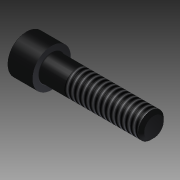
# Autodesk Inventor part: 3071
Saved by Autodesk Inventor 2016 (Build 200138000, 138)
## iProperties
Category: PARTsolutions
Company: 8020
Created: 2016-04-17
Part Number: 3071
Catalog Web Link: www.cadenas.de
Description: 3044, 3048, 3052, 3056, 3057, 3058, 3062, 3067, 3064, 3068, 3071, 3072, 3080, 3081, 3082, 3106, 3110, 3112, 3119, 3122, 3123, 3127, 3129, 3130, 3131, 3132, 3133, 3125, 3124-Socket Head Cap Screws
Vendor: 8020
Document SubType Name: Modeling
Designer: psAdmin
Manufacturer: 8020
Mass: 1.18322 g
Surface Area: 8.777 cm^2
Volume: 1.18322 cm^3
Density: 1 g/cm^3
Material: Generic
Appearance: PSOLRGB-0-0-0
PSOL_IDENT_0: {$CADENAS_DATA\23d-libs\8020\inch\fastening_options\3044.prj},308 {VTYP=3D},{NB=3071},{LINA=3071},{N
PSOL_IDENT_1: N=3044, 3048, 3052, 3056, 3057, 3058, 3062, 3067, 3064, 3068, 3071, 3072, 3080, 3081, 3082, 3106, 31
PSOL_IDENT_2: 10, 3112, 3119, 3122, 3123, 3127, 3129, 3130, 3131, 3132, 3133, 3125, 3124},{DATE=22.08.2012},{GEOMD
PSOL_IDENT_3: ATE=11.05.2012 00:00:00},{VERSION=},{LINEID=60},{LINESUBID=-1},{WBVAR=L}  {NB=3071},{LINA=3071},{KT=
PSOL_IDENT_4: DUMMY},{PN=3071},{FIN=Black Zinc},{THRD=1/4-20},{THRD1=0.2500},{L=1.00000000},{L1=[0.375,0.5,0.625,0
PSOL_IDENT_5: .75,0.875,1,1.25,1.5,2.125,2.5]},{TT=UNC},{A=0.375},{H=0.250},{J=0.18750},{T=0.120},{W=.016},{TH=0.2
PSOL_IDENT_6: 500}
NN: 3044, 3048, 3052, 3056, 3057, 3058, 3062, 3067, 3064, 3068, 3071, 3072, 3080, 3081, 3082, 3106, 3110, 3112, 3119, 3122, 3123, 3127, 3129, 3130, 3131, 3132, 3133, 3125, 3124
NT: Socket Head Cap Screws
NB: 3071
NBSYN: $PN.
LINA: 3071
PN: 3071
FIN: Black Zinc
THRD: 1/4-20
L: 1
A: 0.375
H: 0.250
J: 0.18750
W: .016
SUPPLIER: 8020
ARTICLENO: 3071
BOMINFO: 3071
CREATOR: CADENAS GmbH
Title: 3071
Author: Cadenas PARTsolutions
Comments: Socket Head Cap Screws
Autodesk Inventor part; units mm, degrees
ref_plane "YZ Plane" through (0, 0, 0) normal (1, 0, 0) x (0, 1, 0)
ref_plane "XZ Plane" through (0, 0, 0) normal (0, 1, 0) x (-1, 0, 0)
ref_plane "XY Plane" through (0, 0, 0) normal (0, 0, 1) x (1, 0, 0)
sketch "Sketch_1" plane through (0, 0, 0) normal (0, 0, 1) x (1, 0, 0)
  line L0 (25.4, 0) -> (-6.35, 0)
  line L1 (-6.35, 0) -> (-6.35, 4.572)
  line L2 (-6.35, 4.572) -> (-6.1595, 4.7625)
  line L3 (-6.1595, 4.7625) -> (0, 4.7625)
  line L4 (0, 4.7625) -> (0, 3.3655)
  arc A0 (0, 3.3655) -> (0.1905, 3.175) centre (0.1905, 3.3655) ccw
  line L5 (0.1905, 3.175) -> (24.6443, 3.175)
  line L6 (24.6443, 3.175) -> (25.4, 2.4194)
  line L7 (25.4, 2.4194) -> (25.4, 0)
  line L8 (25.4, 0) -> (-6.35, 0)
  constraints: 18 end point, 2 point on circle, 1 centre point
revolve "Revolution1" add sketch "Sketch_1" angle 360 about axis through (25.4, 0, 0) along (1, 0, 0)
thread "Thread1" size "1/4-20 UNC" class "2A" standard "ANSI Unified Screw Threads" length 18.2943
sketch "Sketch_3" plane through (-6.35, 0, 0) normal (1, 0, 0) x (0, 0, -1)
  line L0 (-2.3813, -1.3748) -> (0, -2.7496)
  line L1 (0, -2.7496) -> (2.3813, -1.3748)
  line L2 (2.3813, -1.3748) -> (2.3813, 1.3748)
  line L3 (2.3813, 1.3748) -> (0, 2.7496)
  line L4 (0, 2.7496) -> (-2.3813, 1.3748)
  line L5 (-2.3813, 1.3748) -> (-2.3813, -1.3748)
  constraints: 12 end point
extrude "Extrusion1" cut sketch "Sketch_3" along normal blind 3.048
sketch "Sketch_4" plane through (0, 0, 0) normal (0, 0, 1) x (1, 0, 0)
  line L0 (-1.9272, 0) -> (-3.302, 0)
  line L1 (-3.302, 0) -> (-3.302, 2.3813)
  line L2 (-3.302, 2.3813) -> (-1.9272, 0)
  line L3 (-1.9272, 0) -> (-3.302, 0)
  constraints: 8 end point
revolve "Revolution2" cut sketch "Sketch_4" angle 360 about axis through (-1.9272, 0, 0) along (1, 0, 0)
ref_plane "screw_XY" through (0, 0, 0) normal (1, 0, 0) x (0, 0, -1)
ref_plane "screw_YZ" through (0, 0, 0) normal (0, 0, -1) x (0, 1, 0)
ref_plane "screw_ZX" through (0, 0, 0) normal (0, 1, 0) x (1, 0, 0)
ref_plane "screw1_XY" through (25.4, 0, 0) normal (1, 0, 0) x (0, 0, -1)
ref_plane "screw1_YZ" through (25.4, 0, 0) normal (0, 0, -1) x (0, 1, 0)
ref_plane "screw1_ZX" through (25.4, 0, 0) normal (0, 1, 0) x (1, 0, 0)
ref_plane "screw2_XY" through (20.32, 0, 0) normal (1, 0, 0) x (0, 0, -1)
ref_plane "screw2_YZ" through (20.32, 0, 0) normal (0, 0, -1) x (0, 1, 0)
ref_plane "screw2_ZX" through (20.32, 0, 0) normal (0, 1, 0) x (1, 0, 0)
ref_plane "to_tnut_XY" through (7.366, 0, 0) normal (1, 0, 0) x (0, 0, -1)
ref_plane "to_tnut_YZ" through (7.366, 0, 0) normal (0, 0, -1) x (0, 1, 0)
ref_plane "to_tnut_ZX" through (7.366, 0, 0) normal (0, 1, 0) x (1, 0, 0)
body "Solid1"
